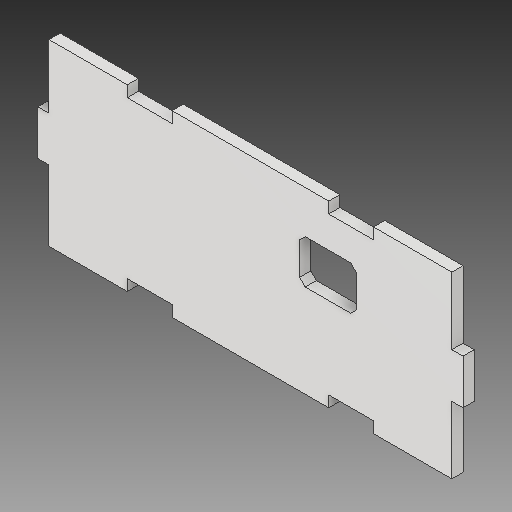
# Autodesk Inventor part: Side 2
Saved by Autodesk Inventor 2018.2 (Build 222227000, 227)
## iProperties
Created: 2018-04-16
Part Number: Side 2
Material: ABS Plastic
Document SubType Name: Modeling
Designer: Derek Fronek
Density: 1.06 g/cm^3
Appearance: Smooth - White
Author: Derek Fronek
Autodesk Inventor part; units mm, degrees
ref_plane "YZ Plane" through (0, 0, 0) normal (1, 0, 0) x (0, 1, 0)
ref_plane "XZ Plane" through (0, 0, 0) normal (0, 1, 0) x (-1, 0, 0)
ref_plane "XY Plane" through (0, 0, 0) normal (0, 0, 1) x (1, 0, 0)
sketch "Sketch1" plane through (0, 0, 0) normal (0, 0, 1) x (1, 0, 0)
  line L0 (22.225, 0) -> (22.225, 3.175) projected
  line L1 (22.225, -47.625) -> (22.225, -44.45) projected
  line L2 (22.225, -44.45) -> (34.925, -44.45) projected
  line L3 (34.925, -44.45) -> (34.925, -47.625) projected
  line L4 (34.925, -47.625) -> (79.375, -47.625) projected
  line L5 (79.375, -47.625) -> (79.375, -44.45) projected
  line L6 (79.375, -44.45) -> (92.075, -44.45) projected
  line L7 (92.075, -44.45) -> (92.075, -47.625) projected
  line L8 (117.475, 3.175) -> (92.075, 3.175) projected
  line L9 (92.075, 3.175) -> (92.075, 0) projected
  line L10 (92.075, 0) -> (79.375, 0) projected
  line L11 (79.375, 0) -> (79.375, 3.175) projected
  line L12 (79.375, 3.175) -> (34.925, 3.175) projected
  line L13 (34.925, 3.175) -> (34.925, 0) projected
  line L14 (34.925, 0) -> (22.225, 0) projected
  line L15 (85.6063, -21.2725) -> (72.708, -21.2725) projected
  line L16 (72.708, -21.2725) -> (71.1205, -19.685) projected
  line L17 (71.1205, -19.685) -> (71.1205, -10.4775) projected
  line L18 (71.1205, -10.4775) -> (72.708, -8.89) projected
  line L19 (72.708, -8.89) -> (85.6063, -8.89) projected
  line L20 (85.6063, -8.89) -> (87.1938, -10.4775) projected
  line L21 (87.1938, -10.4775) -> (87.1938, -19.685) projected
  line L22 (87.1938, -19.685) -> (85.6063, -21.2725) projected
  line L23 (0, 0) -> (0, 3.175) projected
  line L24 (0, 3.175) -> (22.225, 3.175)
  line L25 (0, -27.6225) -> (-3.175, -27.6225)
  line L26 (-3.175, -27.6225) -> (-3.175, -14.9225)
  line L27 (-3.175, -14.9225) -> (0, -14.9225)
  line L28 (3.175, -14.9225) -> (3.175, -27.6225)
  line L29 (3.175, -27.6225) -> (-3.175, -14.9225) construction
  line L30 (-3.175, -27.6225) -> (3.175, -14.9225) construction
  line L31 (0, -47.625) -> (0, -27.6225)
  line L32 (0, -14.9225) -> (0, 3.175)
  line L33 (114.3, 0) -> (114.3, 3.175) projected
  line L34 (92.075, -47.625) -> (114.3, -47.625)
  line L35 (114.3, -28.575) -> (117.475, -28.575)
  line L36 (117.475, -28.575) -> (117.475, -15.875)
  line L37 (117.475, -15.875) -> (114.3, -15.875)
  line L38 (111.125, -15.875) -> (111.125, -28.575)
  line L39 (111.125, -28.575) -> (117.475, -15.875) construction
  line L40 (117.475, -28.575) -> (111.125, -15.875) construction
  line L41 (114.3, -47.625) -> (114.3, -28.575)
  line L42 (114.3, -15.875) -> (114.3, 3.175)
  line L43 (22.225, -47.625) -> (0, -47.625)
  point P0 (0, -21.2725)
  point P1 (114.3, -22.225)
  dimension "d2" = 6.35
  dimension "d3" = 12.7
  dimension "d4" = 6.35
  dimension "d5" = 12.7
  constraints: 38 end point, 4 horizontal, 4 midpoint, 4 parallel, 4 perpendicular, 4 vertical
  measures "d2" distance of L26.end L28.start
  measures "d3" distance of L25.end L26.end
  measures "d4" distance of L38.start L36.end
  measures "d5" distance of L36.end L35.end
extrude "Extrusion1" add sketch "Sketch1" along normal blind 3.175
body "Solid1"
